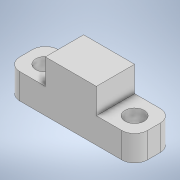
# Autodesk Inventor part: Mirror Feature Practice
Saved by Autodesk Inventor 2020 (Build 240168000, 168)
## iProperties
Created: 2020-02-04
Part Number: Mirror Feature Practice
Material: Generic
Document SubType Name: Modeling
Designer: cks4a449
Density: 1 g/cm^3
Appearance: Default
Author: cks4a449
Autodesk Inventor part; units mm, degrees
ref_plane "YZ Plane" through (0, 0, 0) normal (1, 0, 0) x (0, 1, 0)
ref_plane "XZ Plane" through (0, 0, 0) normal (0, 1, 0) x (-1, 0, 0)
ref_plane "XY Plane" through (0, 0, 0) normal (0, 0, 1) x (1, 0, 0)
sketch "Sketch1" plane through (0, 0, 0) normal (0, 0, 1) x (1, 0, 0)
  line L0 (0, 0) -> (19.05, 0)
  line L1 (19.05, 12.7) -> (0, 12.7)
  line L2 (0, 12.7) -> (0, 0)
  line L3 (19.05, 0) -> (31.75, 0)
  line L4 (31.75, 0) -> (31.75, 25.4)
  line L5 (31.75, 25.4) -> (19.05, 25.4)
  line L6 (19.05, 25.4) -> (19.05, 12.7)
  dimension "d0" = 19.05
  dimension "d2" = 12.7
  dimension "d3" = 25.4
  dimension "d4" = 12.7
  constraints: 14 end point, 3 parallel, 2 horizontal, 1 perpendicular
  measures "d0" distance of L1.start L1.end
  measures "d2" distance of L5.end L4.end
  measures "d3" distance of L4.end L3.end
  measures "d4" distance of L1.end L0.start
extrude "Extrusion1" add sketch "Sketch1" along normal blind 19.05
fillet "Fillet1" radius 6.35 2 edges at (0, 6.35, 19.05) (0, 6.35, 0)
sketch "Sketch2" plane through (19.05, 12.7, 19.05) normal (0, 1, 0) x (1, 0, 0)
  line L0 (0, 19.05) -> (-12.7, 19.05) projected
  line L1 (0, 19.05) -> (0, 0) projected
  circle A0 centre (-9.525, 9.525) radius 4.7625
  line L2 (0, 19.05) -> (-6.1574, 12.8926)
  line L3 (-12.8926, 6.1574) -> (-19.05, 0)
  line L4 (0, 0) -> (-6.1574, 6.1574)
  line L5 (-12.8926, 12.8926) -> (-19.05, 19.05)
  dimension "d8" = 9.525
  constraints: 8 end point, 4 point on circle, 1 centre point
  measures "d8" diameter of A0
extrude "Extrusion2" cut sketch "Sketch2" against normal through all contours A0
mirror "Mirror1" about plane through (31.75, 0, 0) normal (1, 0, 0) of "Extrusion1", "Extrusion2", "Fillet1"
body "Solid1"
